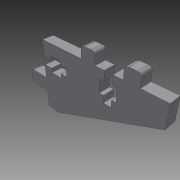
# Autodesk Inventor part: z_axis_top_brace
Saved by Autodesk Inventor 2014 (Build 180170000, 170)
## iProperties
Created: 2014-04-04
Part Number: z_axis_top_brace
Material: Plywood, Finish
Document SubType Name: Modeling
Designer: buben
Density: 0.552 g/cm^3
Appearance: Plywood - New
Author: buben
Autodesk Inventor part; units mm, degrees
ref_plane "YZ Plane" through (0, 0, 0) normal (1, 0, 0) x (0, 1, 0)
ref_plane "XZ Plane" through (0, 0, 0) normal (0, 1, 0) x (-1, 0, 0)
ref_plane "XY Plane" through (0, 0, 0) normal (0, 0, 1) x (1, 0, 0)
sketch "Sketch1" plane through (0, 0, 0) normal (0, 1, 0) x (-1, 0, 0)
  line L0 (0, -40) -> (0, 0)
  line L1 (0, 0) -> (-70, 0)
  line L2 (-70, 0) -> (-70, -12)
  line L3 (-70, -12) -> (-8, -40)
  line L4 (-8, -40) -> (0, -40)
  dimension "d0" = 8
  dimension "d1" = 12
  dimension "d2" = 70
  dimension "d3" = 40
  constraints: 10 end point, 2 parallel, 1 perpendicular, 1 vertical
  measures "d0" distance of L3.end L0.start
  measures "d1" distance of L1.end L2.end
  measures "d2" distance of L0.end L1.end
  measures "d3" distance of L0.start L0.end
extrude "Extrusion1" add sketch "Sketch1" along normal blind 6.5
sketch "Sketch2" plane through (0, 0, 0) normal (0, -1, 0) x (1, 0, 0)
  line L0 (0, 0) -> (0, -40) projected
  line L1 (70, 0) -> (0, 0) projected
  line L2 (39.75, 0) -> (44.25, 0)
  line L3 (44.25, -16.3) -> (39.75, -16.3)
  line L4 (46.75, -5) -> (46.75, -12.3)
  line L5 (37.25, -12.3) -> (37.25, -5)
  line L6 (37.25, -5) -> (39.75, -5)
  line L7 (44.25, -5) -> (46.75, -5)
  line L8 (46.75, -12.3) -> (44.25, -12.3)
  line L9 (39.75, -12.3) -> (37.25, -12.3)
  line L10 (39.75, -16.3) -> (39.75, -12.3)
  line L11 (39.75, -5) -> (39.75, 0)
  line L12 (44.25, 0) -> (44.25, -5)
  line L13 (44.25, -12.3) -> (44.25, -16.3)
  line L14 (0, -13.75) -> (0, -9.25)
  line L15 (16.3, -9.25) -> (16.3, -13.75)
  line L16 (5, -6.75) -> (12.3, -6.75)
  line L17 (12.3, -16.25) -> (5, -16.25)
  line L18 (5, -16.25) -> (5, -13.75)
  line L19 (5, -9.25) -> (5, -6.75)
  line L20 (12.3, -6.75) -> (12.3, -9.25)
  line L21 (12.3, -13.75) -> (12.3, -16.25)
  line L22 (16.3, -13.75) -> (12.3, -13.75)
  line L23 (5, -13.75) -> (0, -13.75)
  line L24 (0, -9.25) -> (5, -9.25)
  line L25 (12.3, -9.25) -> (16.3, -9.25)
  point P0 (42, -16.3)
  point P1 (16.3, -11.5)
  dimension "d6" = 4.5
  dimension "d7" = 4
  dimension "d8" = 5
  dimension "d9" = 7.3
  dimension "d10" = 2.5
  dimension "d11" = 4.5
  dimension "d12" = 4
  dimension "d13" = 5
  dimension "d14" = 7.3
  dimension "d15" = 2.5
  dimension "d16" = 42
  dimension "d17" = 11.5
  constraints: 48 end point, 21 parallel, 12 collinear, 8 perpendicular, 3 horizontal, 2 midpoint
  measures "d6" distance of L3.start L3.end
  measures "d7" distance of L8.end L3.start
  measures "d8" distance of L2.end L7.start
  measures "d9" distance of L4.start L4.end
  measures "d10" distance of L4.end L8.end
  measures "d11" distance of L25.end L22.start
  measures "d12" distance of L20.end L25.end
  measures "d13" distance of L14.end L24.end
  measures "d14" distance of L19.end L16.end
  measures "d15" distance of L16.end L20.end
  measures "d16" distance from line of L0 point (42, -16.3)
  measures "d17" distance from line of L1 point (16.3, -11.5)
extrude "Extrusion2" cut sketch "Sketch2" against normal through all
sketch "Sketch3" plane through (0, 0, 0) normal (0, -1, 0) x (1, 0, 0)
  line L0 (39.75, 0) -> (0, 0) projected
  line L1 (16.3, -9.25) -> (16.3, -13.75) projected
  line L2 (0, -13.75) -> (0, -40) projected
  line L3 (70, 0) -> (44.25, 0) projected
  line L4 (44.25, -16.3) -> (39.75, -16.3) projected
  line L5 (26.5, 0) -> (34.5, 0)
  line L6 (34.5, 0) -> (34.5, 4.5)
  line L7 (32.5, 6.5) -> (28.5, 6.5)
  line L8 (26.5, 4.5) -> (26.5, 0)
  line L9 (49.5, 0) -> (57.5, 0)
  line L10 (57.5, 0) -> (57.5, 4.5)
  line L11 (55.5, 6.5) -> (51.5, 6.5)
  line L12 (49.5, 4.5) -> (49.5, 0)
  line L13 (0, -21.5) -> (-11, -21.5)
  line L14 (-13, -23.5) -> (-13, -27.5)
  line L15 (-11, -29.5) -> (0, -29.5)
  line L16 (0, -29.5) -> (0, -21.5)
  arc A0 (28.5, 6.5) -> (26.5, 4.5) centre (28.5, 4.5) ccw
  arc A1 (34.5, 4.5) -> (32.5, 6.5) centre (32.5, 4.5) ccw
  arc A2 (51.5, 6.5) -> (49.5, 4.5) centre (51.5, 4.5) ccw
  arc A3 (57.5, 4.5) -> (55.5, 6.5) centre (55.5, 4.5) ccw
  arc A4 (-11, -21.5) -> (-13, -23.5) centre (-11, -23.5) ccw
  arc A5 (-13, -27.5) -> (-11, -29.5) centre (-11, -27.5) ccw
  point P0 (16.3, -11.5)
  point P1 (42, -16.3)
  dimension "d20" = 2
  dimension "d21" = 8
  dimension "d22" = 8
  dimension "d23" = 8
  dimension "d24" = 6.5
  dimension "d25" = 15
  dimension "d26" = 13
  dimension "d27" = 7.5
  dimension "d28" = 10
  constraints: 24 end point, 12 point on circle, 12 tangent, 6 centre point, 6 parallel, 5 equal radius, 3 horizontal, 3 perpendicular, 3 point on line, 2 midpoint, 1 collinear
  measures "d20" radius of A0
  measures "d21" distance between parallel lines of L13 L15
  measures "d22" distance between parallel lines of L6 L8
  measures "d23" distance between parallel lines of L10 L12
  measures "d24" distance between parallel lines of L3 L11
  measures "d25" distance between parallel lines of L6 L12
  measures "d26" distance between parallel lines of L2 L14
  measures "d27" distance from line of point (42, -16.3) L6
  measures "d28" distance from line of point (16.3, -11.5) L13
extrude "Extrusion3" add sketch "Sketch3" against normal blind 6.5
equation "\"d22\" = d21"
equation "\"d23\" = d22"
equation "\"d27\" = 0.5 * d25"
body "Solid1"
